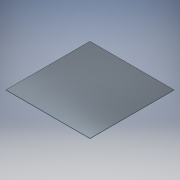
# Autodesk Inventor part: Table
Saved by Autodesk Inventor 2019 (Build 230136000, 136)
## iProperties
Created: 2020-03-19
Part Number: Table
Material: Generic
Document SubType Name: Modeling
Designer: james
Density: 1 g/cm^3
Appearance: Expanded Metal 01
Author: james
Autodesk Inventor part; units mm, degrees
ref_plane "YZ Plane" through (0, 0, 0) normal (1, 0, 0) x (0, 1, 0)
ref_plane "XZ Plane" through (0, 0, 0) normal (0, 1, 0) x (-1, 0, 0)
ref_plane "XY Plane" through (0, 0, 0) normal (0, 0, 1) x (1, 0, 0)
sketch "Sketch1" plane through (0, 0, 0) normal (0, 1, 0) x (-1, 0, 0)
  line L0 (227.6593, 305.1763) -> (-381.9407, 305.1763)
  line L1 (-381.9407, 305.1763) -> (-381.9407, -304.4237)
  line L2 (-381.9407, -304.4237) -> (227.6593, -304.4237)
  line L3 (227.6593, -304.4237) -> (227.6593, 305.1763)
  point P0 (0, 0)
  dimension "d0" = 609.6
  dimension "d1" = 609.6
  constraints: 8 end point, 2 parallel, 1 horizontal, 1 perpendicular
  measures "d0" distance of L2.end L0.start
  measures "d1" distance of L0.start L0.end
extrude "Extrusion1" add sketch "Sketch1" along normal blind 2.54
body "Solid1"
